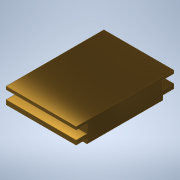
# Autodesk Inventor part: Stamp Body
Saved by Autodesk Inventor 2022 (Build 260153000, 153)
## iProperties
Created: 2021-01-06
Part Number: Stamp Body
Material: Brass
Document SubType Name: Modeling
Designer: caleb
Density: 8.49 g/cm^3
Appearance: Brass - Polished
Author: caleb
Autodesk Inventor part; units mm, degrees
ref_plane "YZ Plane" through (0, 0, 0) normal (1, 0, 0) x (0, 1, 0)
ref_plane "XZ Plane" through (0, 0, 0) normal (0, 1, 0) x (-1, 0, 0)
ref_plane "XY Plane" through (0, 0, 0) normal (0, 0, 1) x (1, 0, 0)
sketch "Sketch1" plane through (0, 0, 0) normal (0, 1, 0) x (-1, 0, 0)
  line L0 (-24, 26) -> (24, 26)
  line L1 (24, 26) -> (24, -26)
  line L2 (24, -26) -> (-24, -26)
  line L3 (-24, -26) -> (-24, 26)
  line L4 (-24, 26) -> (24, -26) construction
  line L5 (24, 26) -> (-24, -26) construction
  point P0 (0, 0)
  dimension "d0" = 52
  dimension "d1" = 48
  constraints: 12 end point, 2 midpoint, 2 parallel, 1 horizontal, 1 perpendicular
  measures "d0" distance of L0.end L1.end
  measures "d1" distance of L1.end L2.end
extrude "Extrusion1" add sketch "Sketch1" along normal blind 14
sketch "Sketch4" plane through (-24, 0, 26) normal (0, 0, 1) x (1, 0, 0)
  line L0 (0, 0) -> (0, 14) projected
  line L1 (48, 0) -> (48, 14) projected
  line L2 (0, 6) -> (48, 6)
  line L3 (48, 6) -> (48, 3)
  line L4 (48, 3) -> (0, 3)
  line L5 (0, 3) -> (0, 6)
  line L6 (0, 14) -> (48, 14) projected
  line L7 (0, 14) -> (48, 14)
  line L8 (48, 14) -> (48, 12)
  line L9 (48, 12) -> (0, 12)
  line L10 (0, 12) -> (0, 14)
  line L11 (48, 0) -> (0, 0) projected
  point P0 (24, 0)
  point P1 (0, 3)
  point P2 (48, 6)
  point P3 (0, 12)
  dimension "d14" = 2
  dimension "d15" = 3
  dimension "d16" = 3
  constraints: 16 end point, 4 parallel, 3 point on line, 2 horizontal, 2 perpendicular
  measures "d14" distance between parallel lines of L6 L9
  measures "d15" distance between parallel lines of L4 L11
  measures "d16" distance between parallel lines of L2 L4
extrude "Extrusion4" add sketch "Sketch4" along normal blind 7.5 contours L0 L2 L1 L4 | L0 L6 L1 L9
sketch "Sketch5" plane through (24, 0, -26) normal (0, 0, -1) x (-1, 0, 0)
  line L0 (0, 6) -> (48, 6)
  line L1 (48, 6) -> (48, 3)
  line L2 (48, 3) -> (0, 3)
  line L3 (0, 3) -> (0, 6)
  line L4 (0, 14) -> (48, 14)
  line L5 (48, 14) -> (48, 12)
  line L6 (48, 12) -> (0, 12)
  line L7 (0, 12) -> (0, 14)
  point P0 (24, 0)
  dimension "d21" = 3
  constraints: 16 end point, 4 parallel, 2 horizontal, 2 perpendicular, 1 point on line
  measures "d21" distance between parallel lines of L0 L2
extrude "Extrusion5" add sketch "Sketch5" along normal blind 7.5
body "Solid1"
